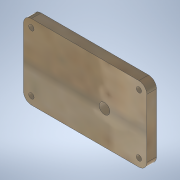
# Autodesk Inventor part: ロボット回転t5.5_2
Saved by Autodesk Inventor 2020.3 (Build 243373000, 373)
## iProperties
Created: 2020-07-07
Part Number: ロボット回転t5.5_2
Material: 木材 (カエデ材)
Document SubType Name: Modeling
Designer: totot
Density: 0.67 g/cm^3
Appearance: ナチュラル カエデ材 - 光沢 濃い着色
Author: totot
Autodesk Inventor part; units mm, degrees
ref_plane "YZ Plane" through (0, 0, 0) normal (1, 0, 0) x (0, 1, 0)
ref_plane "XZ Plane" through (0, 0, 0) normal (0, 1, 0) x (-1, 0, 0)
ref_plane "XY Plane" through (0, 0, 0) normal (0, 0, 1) x (1, 0, 0)
sketch "スケッチ1" plane through (0, 0, 0) normal (0, 0, 1) x (1, 0, 0)
  line L0 (0, 0) -> (70, 0)
  line L1 (70, 0) -> (70, -42.5)
  line L2 (70, -42.5) -> (0, -42.5)
  line L3 (0, -42.5) -> (0, 0)
  dimension "d0" = 70
  dimension "d1" = 42.5
  constraints: 8 end point, 2 parallel, 1 horizontal, 1 perpendicular
  measures "d0" distance of L1.end L2.end
  measures "d1" distance of L0.end L1.end
extrude "押し出し1" add sketch "スケッチ1" along normal blind 5.5
sketch "スケッチ2" plane through (0, 0, 5.5) normal (0, 0, 1) x (1, 0, 0)
  line L0 (4.5, -38) -> (65.5, -38)
  line L1 (65.5, -38) -> (65.5, -4.5)
  line L2 (65.5, -4.5) -> (4.5, -4.5)
  line L3 (4.5, -4.5) -> (4.5, -38)
  line L4 (0, 0) -> (0, -42.5) projected
  line L5 (0, -42.5) -> (70, -42.5) projected
  dimension "d4" = 61
  dimension "d5" = 33.5
  dimension "d6" = 4.5
  dimension "d7" = 4.5
  constraints: 8 end point, 4 coincident, 2 parallel, 1 horizontal, 1 perpendicular
  measures "d4" distance of L2.end L1.end
  measures "d5" distance of L1.end L0.end
  measures "d6" distance between parallel lines of L3 L4
  measures "d7" distance between parallel lines of L0 L5
hole "穴1" at (4.5, -38, 5.5) at (4.5, -4.5, 5.5) at (65.5, -4.5, 5.5) at (65.5, -38, 5.5) direction (0, 0, -1) diameter 3 end through all
fillet "フィレット1" radius 4.5 4 edges at (0, 0, 2.75) (70, 0, 2.75) (70, -42.5, 2.75) (0, -42.5, 2.75)
sketch "スケッチ3" plane through (0, 0, 5.5) normal (0, 0, 1) x (1, 0, 0)
  line L0 (65.5, 0) -> (4.5, 0) projected
  line L1 (70, -38) -> (70, -4.5) projected
  point P0 (0, 0)
  point P1 (46, -23.5)
  dimension "d16" = 23.5
  dimension "d17" = 24
  measures "d16" distance from line of point (46, -23.5) L0
  measures "d17" distance from line of point (46, -23.5) L1
hole "穴2" at (46, -23.5, 5.5) direction (0, 0, -1) diameter 17 end through all
sketch "スケッチ4" plane through (0, 0, 0) normal (0, 0, -1) x (-1, 0, 0)
  line L0 (-4.5, -42.5) -> (-65.5, -42.5) projected
  line L1 (0, -4.5) -> (0, -38) projected
  point P0 (0, 0)
  point P1 (-10, -35.5)
  point P2 (-10, -30)
  point P3 (-10, -24.5)
  point P4 (-10, -19)
  point P5 (-10, -13.5)
  point P6 (-10, -8)
  point P7 (-15.5, -35.5)
  point P8 (-15.5, -30)
  point P9 (-15.5, -24.5)
  point P10 (-15.5, -19)
  point P11 (-15.5, -13.5)
  point P12 (-15.5, -8)
  point P13 (-21, -35.5)
  point P14 (-21, -30)
  point P15 (-21, -24.5)
  point P16 (-21, -19)
  point P17 (-21, -13.5)
  point P18 (-21, -8)
  point P19 (-26.5, -35.5)
  point P20 (-26.5, -30)
  point P21 (-26.5, -24.5)
  point P22 (-26.5, -19)
  point P23 (-26.5, -13.5)
  point P24 (-26.5, -8)
  point P25 (-32, -35.5)
  point P26 (-32, -30)
  point P27 (-32, -24.5)
  point P28 (-32, -19)
  point P29 (-32, -13.5)
  point P30 (-32, -8)
  dimension "d25" = 7
  dimension "d26" = 10
  dimension "d29" = 5.5
  dimension "d32" = 5.5
  constraints: 1 horizontal, 1 vertical, 29 other
  measures "d25" distance from line of L0 point (-10, -35.5)
  measures "d26" distance from line of L1 point (-10, -35.5)
  measures "d29" distance of point (-10, -35.5) point (-10, -30)
  measures "d32" distance of point (-10, -35.5) point (-15.5, -35.5)
hole "穴3" at (10, -35.5, 0) at (10, -30, 0) at (10, -24.5, 0) at (10, -19, 0) at (10, -13.5, 0) at (10, -8, 0) at (15.5, -35.5, 0) at (15.5, -30, 0) at (15.5, -24.5, 0) at (15.5, -19, 0) at (15.5, -13.5, 0) at (15.5, -8, 0) at (21, -35.5, 0) at (21, -30, 0) at (21, -24.5, 0) at (21, -19, 0) at (21, -13.5, 0) at (21, -8, 0) at (26.5, -35.5, 0) at (26.5, -30, 0) at (26.5, -24.5, 0) at (26.5, -19, 0) at (26.5, -13.5, 0) at (26.5, -8, 0) at (32, -35.5, 0) at (32, -30, 0) at (32, -24.5, 0) at (32, -19, 0) at (32, -13.5, 0) at (32, -8, 0) direction (0, 0, 1) diameter 4.5 end through all
